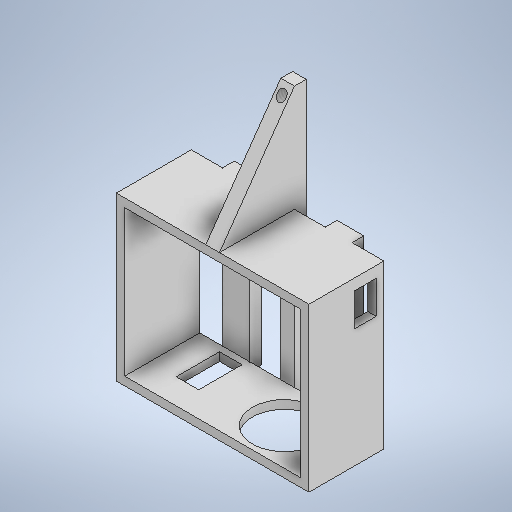
# Autodesk Inventor part: SENX_Mount
Saved by Autodesk Inventor 2025 (Build 290162010, 162A)
## iProperties
Created: 2024-06-25
Part Number: SENX_Mount
Material: Generic
Document SubType Name: Modeling
Designer: vncnt
Density: 1 g/cm^3
Appearance: Default
Author: vncnt
Autodesk Inventor part; units mm, degrees
ref_plane "YZ Plane" through (0, 0, 0) normal (1, 0, 0) x (0, 1, 0)
ref_plane "XZ Plane" through (0, 0, 0) normal (0, 1, 0) x (-1, 0, 0)
ref_plane "XY Plane" through (0, 0, 0) normal (0, 0, 1) x (1, 0, 0)
sketch "Sketch1" plane through (0, 0, 0) normal (0, 0, 1) x (1, 0, 0)
  line L0 (26.15, 21.71) -> (26.15, -21.71)
  line L1 (-26.15, 21.71) -> (26.15, -21.71) construction
  line L2 (26.15, 21.71) -> (-26.15, -21.71) construction
  line L3 (28.65, -24.21) -> (28.65, 24.21)
  line L4 (-17.6647, 24.21) -> (11.8813, -16.2837) construction
  line L5 (22, 17) -> (-22, -17) construction
  line L6 (22, -24.21) -> (28.65, -24.21)
  line L7 (26.15, -21.71) -> (22, -21.71)
  line L8 (22, -21.71) -> (22, -24.21)
  line L9 (0, 21.71) -> (0, 40)
  line L10 (28.65, 24.21) -> (0, 24.21)
  line L11 (0, 21.71) -> (26.15, 21.71)
  line L12 (-26.15, 21.71) -> (-26.15, -21.71)
  line L13 (-28.65, -24.21) -> (-28.65, 24.21)
  line L14 (-22, -24.21) -> (-28.65, -24.21)
  line L15 (-26.15, -21.71) -> (-22, -21.71)
  line L16 (-22, -21.71) -> (-22, -24.21)
  line L17 (-28.65, 24.21) -> (0, 24.21)
  line L18 (0, 21.71) -> (-26.15, 21.71)
  line L19 (-22, -21.71) -> (22, -21.71)
  line L20 (22, -21.71) -> (22, -24.21)
  line L21 (22, -24.21) -> (-22, -24.21)
  line L22 (-22, -24.21) -> (-22, -21.71)
  point P0 (0, 0)
  point P1 (-11.8813, -16.2837)
  point P2 (-22, 17)
  dimension "d1" = 43.42
  dimension "d21" = 28.65
  dimension "d22" = 26.15
  constraints: 46 end point, 6 symmetric about line, 4 parallel, 3 midpoint, 3 perpendicular, 2 horizontal, 2 point on line, 1 vertical
  measures "d1" distance of L0.start L0.end
  measures "d21" distance between parallel lines of L3 L9
  measures "d22" distance of L9.start L0.start
extrude "Extrusion1" add sketch "Sketch1" along normal blind 22.3 contours L11 L9 L10 L3 L6 L8 L7 L0 | L18 L12 L15 L16 L14 L13 L17 L9 | L8 L21 L16 L19
sketch "Sketch4" plane through (-28.65, 24.21, 0) normal (0, 1, 0) x (1, 0, 0)
  line L0 (26.618, -3.5) -> (30.682, -3.5)
  line L1 (30.682, -3.5) -> (30.682, 3.5)
  line L2 (30.682, 3.5) -> (26.618, 3.5)
  line L3 (26.618, 3.5) -> (26.618, -3.5)
  line L4 (26.618, -3.5) -> (30.682, 3.5) construction
  line L5 (30.682, -3.5) -> (26.618, 3.5) construction
  line L6 (57.3, 0) -> (0, 0) projected
  line L7 (25.7756, 0) -> (33, 0)
  point P0 (28.65, 0)
  point P1 (26.618, 0)
  point P2 (30.682, 0)
  dimension "d23" = 4.064
  dimension "d24" = 7
  constraints: 14 end point, 2 midpoint, 2 parallel, 1 horizontal, 1 perpendicular, 1 point on line
  measures "d23" distance of L2.end L1.end
  measures "d24" distance of L1.end L0.end
extrude "Extrusion3" add sketch "Sketch4" along normal blind 31.75 and the other way blind 48.42 contours L3 L2 L1 L6
sketch "Sketch6" plane through (28.65, -24.21, 0) normal (1, 0, 0) x (0, 0, -1)
  line L0 (-8.7, 45.12) -> (-2.3, 45.12)
  line L1 (-2.3, 45.12) -> (-2.3, 35.32)
  line L2 (-2.3, 35.32) -> (-8.7, 35.32)
  line L3 (-8.7, 35.32) -> (-8.7, 45.12)
  line L4 (-8.7, 45.12) -> (-2.3, 35.32) construction
  line L5 (-2.3, 45.12) -> (-8.7, 35.32) construction
  line L6 (0, 0) -> (0, 48.42) projected
  line L7 (0, 48.42) -> (-22.3, 48.42) projected
  point P0 (0, 24.21)
  point P1 (-5.5, 40.22)
  dimension "d38" = 6.4
  dimension "d39" = 9.8
  dimension "d40" = 2.3
  dimension "d41" = 3.3
  constraints: 12 end point, 2 midpoint, 2 parallel, 1 horizontal, 1 perpendicular
  measures "d38" distance of L1.end L2.end
  measures "d39" distance of L0.end L1.end
  measures "d40" distance between parallel lines of L6 L1
  measures "d41" distance between parallel lines of L7 L0
extrude "Extrusion4" cut sketch "Sketch6" against normal blind 20
sketch "Sketch7" plane through (2.032, -24.21, -3.5) normal (1, 0, 0) x (0, 0, -1)
  line L0 (0, 80.17) -> (-3.5, 80.17) projected
  line L1 (-3.5, 48.42) -> (-25.8, 48.42) projected
  line L2 (-3.5, 80.17) -> (-25.8, 80.17)
  line L3 (-25.8, 80.17) -> (-25.8, 48.42)
  line L4 (-25.8, 48.42) -> (-3.5, 48.42)
  line L5 (-3.5, 48.42) -> (-3.5, 80.17)
  line L6 (-25.8, 48.42) -> (-3.5, 80.17)
  point P0 (-3.5, 24.21)
  constraints: 10 end point, 2 parallel, 1 horizontal, 1 perpendicular
extrude "Extrusion5" add sketch "Sketch7" against normal up to surface (4.064 mm away) contours L1 L6 L5
sketch "Sketch8" plane through (2.032, 55.96, -3.5) normal (0, 0, -1) x (-1, 0, 0)
  line L0 (0, 0) -> (4.064, 0) projected
  line L1 (0, -80.17) -> (0, 0) projected
  point P0 (2.032, -55.96)
  point P1 (2.032, -2.5)
  dimension "d46" = 2.5
  dimension "d47" = 2.032
  measures "d46" distance from line of L0 point (2.032, -2.5)
  measures "d47" distance from line of L1 point (2.032, -2.5)
hole "Hole3" at (0, 53.46, -3.5) direction (0, 0, 1) diameter 2.6416 depth 10.979 thread size "6-32 UNC" class "2B" standard "ANSI Unified Screw Threads"
sketch "Sketch10" plane through (-28.65, -24.21, 22.3) normal (0, -1, 0) x (1, 0, 0)
  circle A0 centre (39, -11) radius 9.5
  line L0 (10.306, -7.5) -> (17.006, -7.5)
  line L1 (17.006, -7.5) -> (17.006, -20.4)
  line L2 (17.006, -20.4) -> (10.306, -20.4)
  line L3 (10.306, -20.4) -> (10.306, -7.5)
  line L4 (57.3, -22.3) -> (57.3, 0) projected
  line L5 (30.682, -22.3) -> (57.3, -22.3) projected
  line L6 (0, -22.3) -> (26.618, -22.3) projected
  point P0 (28.65, -22.3)
  point P1 (43.991, -22.3)
  dimension "d59" = 18.3
  dimension "d60" = 11.3
  dimension "d61" = 19
  dimension "d62" = 6.7
  dimension "d63" = 12.9
  dimension "d64" = 40.294
  dimension "d65" = 1.9
  constraints: 8 end point, 2 parallel, 1 centre point, 1 horizontal, 1 midpoint, 1 perpendicular
  measures "d59" distance from line of L4 A0.centre
  measures "d60" vertical distance of point (43.991, -22.3) A0.centre
  measures "d61" diameter of A0
  measures "d62" distance of L1.end L2.end
  measures "d63" distance of L0.end L1.end
  measures "d64" distance between parallel lines of L4 L1
  measures "d65" distance between parallel lines of L6 L2
extrude "Extrusion7" cut sketch "Sketch10" against normal blind 31.75
sketch "Sketch12" plane through (28.65, 24.21, 22.3) normal (0, 1, 0) x (1, 0, 0)
  line L0 (-2.5, 22.3) -> (-26.618, 22.3) projected
  line L1 (-16.2, 22.3) -> (-17, 22.3)
  line L2 (-54.8, 22.3) -> (-30.682, 22.3) projected
  line L3 (-41, 22.3) -> (-46.5768, 22.3)
  line L4 (-48, 22.3) -> (-39.837, 22.3)
  line L5 (-39.837, 22.3) -> (-39.837, 25.8)
  line L6 (-39.837, 25.8) -> (-48, 25.8)
  line L7 (-48, 25.8) -> (-48, 22.3)
  line L8 (-17.463, 22.3) -> (-9.463, 22.3)
  line L9 (-9.463, 22.3) -> (-9.463, 25.8)
  line L10 (-9.463, 25.8) -> (-17.463, 25.8)
  line L11 (-17.463, 25.8) -> (-17.463, 22.3)
  line L12 (-30.682, 25.8) -> (-30.682, 22.3) projected
  line L13 (-26.618, 22.3) -> (-26.618, 25.8) projected
  point P0 (-28.65, 22.3)
  point P1 (-9.463, 22.3)
  dimension "d69" = 8
  dimension "d70" = 3.5
  dimension "d71" = 3.5
  dimension "d72" = 9.155
  dimension "d73" = 9.155
  constraints: 20 end point, 4 parallel, 4 point on line, 3 horizontal, 2 perpendicular
  measures "d69" distance of L10.end L9.end
  measures "d70" distance of L4.end L5.end
  measures "d71" distance of L8.end L9.end
  measures "d72" distance between parallel lines of L12 L5
  measures "d73" distance between parallel lines of L13 L11
extrude "Extrusion8" add sketch "Sketch12" against normal up to surface (48.42 mm away)
body "Solid1"
